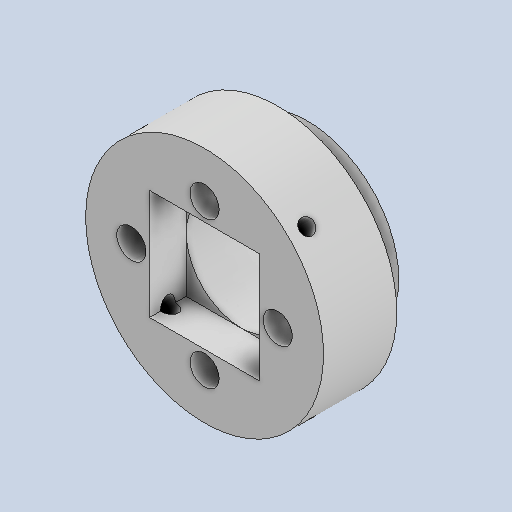
# Autodesk Inventor part: bearing_bracket4
Saved by Autodesk Inventor 2026.1 (Build 301233000, 233)
## iProperties
Created: 2026-04-12
Part Number: bearing_bracket4
Material: Generic
Document SubType Name: Modeling
Designer: chris
Density: 1 g/cm^3
Appearance: Default
Author: chris
Autodesk Inventor part; units mm, degrees
ref_plane "YZ Plane" through (0, 0, 0) normal (1, 0, 0) x (0, 1, 0)
sketch "Sketch1" plane through (0, 0, 0) normal (0, 0, 1) x (1, 0, 0)
  circle A0 centre (0, 0) radius 24.95
  dimension "d0" = 49.9
  constraints: 1 centre point, 1 coincident
  measures "d0" diameter of A0
extrude "Extrusion1" add sketch "Sketch1" along normal blind 8.1
sketch "Sketch2" plane through (0, 0, 8.1) normal (0, 0, 1) x (1, 0, 0)
  circle A0 centre (0, 0) radius 15
  dimension "d3" = 30
  constraints: 1 centre point, 1 coincident
  measures "d3" diameter of A0
extrude "Extrusion2" cut sketch "Sketch2" against normal through all
sketch "Sketch3" plane through (0, 0, 8.1) normal (0, 0, 1) x (1, 0, 0)
  circle A0 centre (0, 0) radius 15
  circle A1 centre (0, 0) radius 32.5
  dimension "d6" = 30
  dimension "d7" = 65
  constraints: 2 centre point, 2 coincident
  measures "d6" diameter of A0
  measures "d7" diameter of A1
extrude "Extrusion3" add sketch "Sketch3" along normal blind 20
sketch "Sketch5" plane through (0, 0, 28.1) normal (0, 0, 1) x (1, 0, 0)
  line L0 (-15.05, -15.05) -> (15.05, -15.05)
  line L1 (15.05, -15.05) -> (15.05, 15.05)
  line L2 (15.05, 15.05) -> (-15.05, 15.05)
  line L3 (-15.05, 15.05) -> (-15.05, -15.05)
  line L4 (-15.05, -15.05) -> (15.05, 15.05) construction
  line L5 (15.05, -15.05) -> (-15.05, 15.05) construction
  point P0 (0, 0)
  dimension "d11" = 30.1
  dimension "d12" = 30.1
  constraints: 12 end point, 2 midpoint, 2 parallel, 1 horizontal, 1 perpendicular
  measures "d11" distance of L2.end L1.end
  measures "d12" distance of L1.end L0.end
extrude "Extrusion4" cut sketch "Sketch5" against normal blind 10
sketch "Sketch6" plane through (0, 0, 0) normal (0, 0, -1) x (-1, 0, 0)
  circle A0 centre (0, 20) radius 2.05 projected
  circle A1 centre (-20, 0) radius 2.05 projected
  circle A2 centre (20, 0) radius 2.05 projected
  circle A3 centre (0, -20) radius 2.05 projected
  point P0 (0, 0)
hole "Hole1" at (20, 0, 0) at (0, 20, 0) at (0, -20, 0) at (-20, 0, 0) direction (0, 0, 1) diameter 4.1 end through all
sketch "Sketch7" plane through (0, 0, 28.1) normal (0, 0, 1) x (1, 0, 0)
  circle A0 centre (20, 0) radius 2.05 projected
  circle A1 centre (0, -20) radius 2.05 projected
  circle A2 centre (-20, 0) radius 2.05 projected
  circle A3 centre (0, 20) radius 2.05 projected
  circle A4 centre (20, 0) radius 4
  circle A5 centre (0, -20) radius 4
  circle A6 centre (-20, 0) radius 4
  circle A7 centre (0, 20) radius 4
  point P0 (0, 0)
  dimension "d22" = 8
  dimension "d23" = 8
  dimension "d24" = 8
  dimension "d25" = 8
  constraints: 4 centre point, 4 coincident
  measures "d22" diameter of A4
  measures "d23" diameter of A5
  measures "d24" diameter of A6
  measures "d25" diameter of A7
extrude "Extrusion5" cut sketch "Sketch7" against normal blind 15 contours A0 | A1 | A2 | A3 | A4 | A5 | A6 | A7
ref_plane "Work Plane1" through (-15.05, -15.05, 28.1) normal (0.7071, -0.7071, 0) x (0, 0, -1)
ref_plane "Work Plane2" through (15.05, -15.05, 28.1) normal (0.7071, 0.7071, 0) x (0, 0, -1)
sketch "Sketch8" plane through (-15.05, -15.05, 28.1) normal (0.7071, -0.7071, 0) x (0, 0, -1)
  spline S0 degree 3 poles (5, 23.3339) (4.7425, 23.3339) (4.4679, 23.2824) (3.9629, 23.0732) (3.7324, 22.9155) (3.3685, 22.5515) (3.2107, 22.321) (3.0015, 21.816) (2.95, 21.5414) (2.95, 21.0264) (3.0015, 20.7518) (3.2107, 20.2468) (3.3685, 20.0163) (3.7324, 19.6524) (3.9629, 19.4946) (4.4679, 19.2854) (4.7425, 19.2339) (5.2575, 19.2339) (5.5321, 19.2854) (6.0371, 19.4946) (6.2676, 19.6524) (6.6315, 20.0163) (6.7893, 20.2468) (6.9985, 20.7518) (7.05, 21.0264) (7.05, 21.5414) (6.9985, 21.816) (6.7893, 22.321) (6.6315, 22.5515) (6.2676, 22.9155) (6.0371, 23.0732) (5.5321, 23.2824) (5.2575, 23.3339) (5, 23.3339) knots 0 0 0 0 0.077243 0.077243 0.154485 0.154485 0.231728 0.231728 0.30897 0.30897 0.386212 0.386212 0.463455 0.463455 0.540697 0.540697 0.61794 0.61794 0.695183 0.695183 0.772425 0.772425 0.849668 0.849668 0.92691 0.92691 1.004153 1.004153 1.081395 1.081395 1.158638 1.158638 1.23588 1.23588 1.23588 1.23588 projected
  point P0 (28.1, 21.2839)
  point P1 (5, 23.3339)
extrude "Extrusion6" cut sketch "Sketch8" along normal through all both and the other way through all
sketch "Sketch9" plane through (15.05, -15.05, 28.1) normal (0.7071, 0.7071, 0) x (0, 0, -1)
  circle A0 centre (5, 21.2839) radius 2.05 projected
  point P0 (28.1, 21.2839)
extrude "Extrusion7" cut sketch "Sketch9" along normal through all both and the other way through all
body "Solid1"
